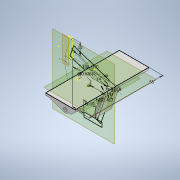
# Autodesk Inventor part: Capping_RotationAnchor
Saved by Autodesk Inventor 2022 (Build 260153000, 153)
## iProperties
Created: 2024-05-05
Part Number: Capping_RotationAnchor
Material: Generic
Document SubType Name: Modeling
Designer: raphael.hauk
Density: 1 g/cm^3
Appearance: Default
Author: raphael.hauk
Autodesk Inventor part; units mm, degrees
ref_plane "YZ Plane" through (0, 0, 0) normal (1, 0, 0) x (0, 1, 0)
ref_plane "XZ Plane" through (0, 0, 0) normal (0, 1, 0) x (-1, 0, 0)
ref_plane "XY Plane" through (0, 0, 0) normal (0, 0, 1) x (1, 0, 0)
ref_plane "Work Plane6" through (7.98, 0, 4.3086) normal (0, 0, 1) x (1, 0, 0)
sketch "Sketch1" plane through (0, 0, 0) normal (0, 0, 1) x (1, 0, 0)
  line L0 (7.98, 8) -> (7.98, -8) projected
  line L1 (7.98, 8) -> (3.98, 8) projected
  line L2 (3.98, -8) -> (3.98, 8) projected
  line L3 (7.98, -8) -> (3.98, -8) projected
  point P0 (0, 0)
  point P1 (21.25, -8.826)
  constraints: 2 other
sketch "Sketch2" plane through (0, 0, 0) normal (0, 0, 1) x (1, 0, 0)
  line L0 (17.98, -43.252) -> (33.98, -43.252)
  line L1 (33.98, -43.252) -> (33.98, -47.252)
  line L2 (33.98, -47.252) -> (17.98, -47.252)
  line L3 (17.98, -47.252) -> (17.98, -43.252)
  line L4 (3.98, -8) -> (3.98, 8) construction
  line L5 (7.98, 8) -> (3.98, 8) construction
  line L6 (7.98, 8) -> (7.98, -8) construction
  line L7 (7.98, -8) -> (3.98, -8) construction
  line L8 (38.606, -12.626) -> (7.98, -2) construction
  line L9 (27.98, -43.252) -> (38.606, -12.626) construction
  arc A0 (7.98, 8) -> (17.98, -43.252) centre (38.606, -12.626) ccw construction
  line L10 (21.25, -8.826) -> (0, -8.826) construction
  line L11 (8.9996, 2.9386) -> (40.245, -7.9022)
  line L12 (40.245, -7.9022) -> (36.967, -17.3498)
  line L13 (36.967, -17.3498) -> (5.7217, -6.5089)
  line L14 (5.7217, -6.5089) -> (8.9996, 2.9386)
  line L15 (8.9996, 2.9386) -> (36.967, -17.3498) construction
  line L16 (40.245, -7.9022) -> (5.7217, -6.5089) construction
  line L17 (38.606, -12.626) -> (27.98, -43.252)
  line L18 (27.98, -43.252) -> (32.7038, -44.891)
  line L19 (32.7038, -44.891) -> (43.3298, -14.265)
  line L20 (43.3298, -14.265) -> (38.606, -12.626)
  point P0 (34.0169, -25.8525)
  point P1 (25.3795, -8.0369)
  point P2 (22.9833, -7.2056)
  point P3 (7.98, 0)
  dimension "d0" = 10
  dimension "d3" = 10
  dimension "d5" = 10
  dimension "d6" = 32.417
  dimension "d7" = 32.417
  dimension "d8" = 3.8
  dimension "d9" = 30.626
  dimension "d26" = 14
  dimension "d27" = 14
  dimension "d44" = 10
  dimension "d47" = 5
  constraints: 34 end point, 7 parallel, 6 point on line, 5 perpendicular, 4 midpoint, 2 horizontal, 2 point on circle, 1 centre point, 1 coincident, 1 collinear
  measures "d0" distance between parallel lines of L3 L6
  measures "d3" distance of L5.start L8.end
  measures "d5" distance of L0.start L9.start
  measures "d6" distance of L8.start L8.end
  measures "d7" distance of L9.start L8.start
  measures "d8" distance from line of L17.start L10
  measures "d9" distance from line of L6 L17.start
  measures "d26" distance of point (25.379, -8.037) L17.start
  measures "d27" distance of point (34.017, -25.853) L17.start
  measures "d44" distance of L11.end L12.end
  measures "d47" distance of L19.end L17.start
ref_plane "Work Plane1" through (18.228, -8.826, 23.9001) normal (0, -1, 0) x (0, 0, -1)
sketch "Sketch3" plane through (18.228, -8.826, 23.9001) normal (0, -1, 0) x (0, 0, -1)
  circle A0 centre (11.5, 16.822) radius 1.45 construction
  circle A1 centre (26.5, 16.822) radius 1.45 construction
  circle A2 centre (11.5, 6.822) radius 1.45 construction
  circle A3 centre (26.5, 6.822) radius 1.45 construction
  line L0 (-12.9085, 2.822) -> (52.0915, 2.822)
  line L1 (52.0915, 2.822) -> (52.0915, 28.822)
  line L2 (52.0915, 28.822) -> (-12.9085, 28.822)
  line L3 (-12.9085, 28.822) -> (-12.9085, 2.822)
  line L4 (19.5915, -18.302) -> (19.5915, 38.076) construction
  point P0 (23.9001, -18.228)
  dimension "d10" = 12
  dimension "d11" = 4
  dimension "d55" = 65
  constraints: 10 end point, 2 parallel, 1 horizontal, 1 perpendicular, 1 vertical, 3 other
  measures "d10" distance from line of L2 A0.centre
  measures "d11" distance from line of L0 A2.centre
  measures "d55" distance of L1.end L2.end
extrude "Extrusion1" add sketch "Sketch3" along normal blind 2
ref_plane "Work Plane3" through (18.228, -12.826, 23.9001) normal (0, -1, 0) x (1, 0, 0)
sketch "Sketch4" plane through (18.228, -12.826, 23.9001) normal (0, -1, 0) x (1, 0, 0)
  point P0 (-18.228, -23.9001)
  point P1 (6.822, -11.5)
  point P2 (6.822, -26.5)
  point P3 (16.822, -11.5)
  point P4 (16.822, -26.5)
sketch "Sketch5" plane through (29.03, -8.826, 4.3086) normal (0, 0, 1) x (1, 0, 0)
  circle A0 centre (9.576, -3.8) radius 1.5
  line L0 (-7.98, -2) -> (18.02, -2) projected
  arc A1 (8.5926, -6.6343) -> (12.4266, -4.7349) centre (9.576, -3.8) ccw
  line L1 (7.937, -8.5238) -> (-23.3083, 2.3171) construction
  line L2 (7.937, -8.5238) -> (-8.6356, -2.7737) construction
  line L3 (-8.6356, -2.7737) -> (-7.98, -0.8842) construction
  line L4 (-7.98, -0.8842) -> (8.5926, -6.6343) construction
  line L5 (8.5926, -6.6343) -> (7.937, -8.5238) construction
  line L6 (-7.98, -2) -> (-7.98, -0.8842)
  line L7 (-7.98, -0.8842) -> (8.5926, -6.6343)
  line L8 (3.6738, -36.065) -> (14.2998, -5.439) construction
  line L9 (14.2998, -5.439) -> (8.5497, -22.0116) construction
  line L10 (8.5497, -22.0116) -> (6.6602, -21.356) construction
  line L11 (6.6602, -21.356) -> (12.4103, -4.7834) construction
  line L12 (12.4103, -4.7834) -> (14.2998, -5.439)
  arc A2 (8.5926, -6.6343) -> (12.4103, -4.7834) centre (9.576, -3.8) ccw construction
  line L13 (14.2998, -5.439) -> (18.02, -2)
  point P0 (-29.03, 8.826)
  point P1 (12.4103, -4.7834)
  point P2 (-4.7641, -2)
  dimension "d21" = 3
  dimension "d46" = 2
  constraints: 22 end point, 5 equal length, 4 perpendicular, 4 point on circle, 4 point on line, 3 centre point, 3 coincident, 1 tangent, 1 vertical
  measures "d21" diameter of A0
  measures "d46" distance between parallel lines of L1 L4
extrude "Extrusion2" add sketch "Sketch5" along normal mid plane 65 contours L0 L13 L12 A1 L7
ref_plane "Work Plane5" through (47.05, -8.826, 4.3086) normal (0, 0, -1) x (-1, 0, 0)
sketch "Sketch7" plane through (47.05, -8.826, 4.3086) normal (0, 0, -1) x (-1, 0, 0)
  line L0 (0, -2) -> (7.4703, -22.7055)
  line L1 (7.4703, -22.7055) -> (9.4703, -22.0116)
  line L2 (3.7202, -5.439) -> (9.4703, -22.0116) construction
  line L3 (0, 0) -> (0, -2) construction
  line L4 (0, -2) -> (3.7202, -5.439)
  line L5 (9.4703, -22.0116) -> (3.7202, -5.439)
  line L6 (0, -2) -> (3.7202, -5.439) projected
  line L7 (0, -2) -> (0, -7.9648)
  line L8 (0, -7.9648) -> (7.4703, -22.7055)
  point P0 (47.05, 8.826)
  point P1 (0, -2)
  dimension "d51" = 2
  constraints: 12 end point, 1 coincident, 1 collinear, 1 perpendicular, 1 vertical
  measures "d51" horizontal distance of L0.end L1.end
extrude "Extrusion3" add sketch "Sketch7" along normal mid plane 14 contours L4 L5 L1 L0
hole "Hole1" at (35.05, -12.826, 12.4001) at (35.05, -12.826, -2.5999) direction (0, 1, 0) diameter 2.6 end through all start extended yes counterbore diameter 5.5 counterbore depth 2 clearance for "Socket Head Cap Screw ISO 4762" size "M2.5" standard "ISO"
fillet "Fillet1" radius 1 2 edges at (45.1899, -12.5455, 11.3086) (45.1899, -12.5455, -2.6914)
sketch "Sketch8" plane through (37.6226, -15.4603, -28.1914) normal (-0.3277907, -0.9447504, 0) x (0.9447504, -0.3277907, 0)
  circle A0 centre (-8, 32.5) radius 5
  line L0 (32.3377, 32.5) -> (-58.7333, 32.5) projected
  line L1 (0, 26.5631) -> (0, 39.6199) projected
  point P0 (-40.6117, 28.1914)
  dimension "d56" = 10
  dimension "d57" = 8
  constraints: 1 centre point, 1 point on line
  measures "d56" diameter of A0
  measures "d57" distance from line of A0.centre L1
extrude "Extrusion4" cut sketch "Sketch8" against normal blind 1
sketch "Sketch9" plane through (37.5797, -30.8376, -2.6914) normal (-0.9447504, 0.3277907, 0) x (0, 0, 1)
  circle A0 centre (7, 9.5418) radius 5
  line L0 (7, -42.3865) -> (7, 53.4932) projected
  line L1 (15, 17.5418) -> (-1, 17.5418) projected
  point P0 (2.6914, 16.8155)
  dimension "d60" = 10
  dimension "d61" = 8
  constraints: 1 centre point, 1 point on line
  measures "d60" diameter of A0
  measures "d61" distance from line of A0.centre L1
extrude "Extrusion5" cut sketch "Sketch9" against normal blind 1
equation "\"d5\" = d3"
equation "\"d7\" = d6"
equation "\"d27\" = d26"
equation "\"d47\" = 0.5 * d44"
body "Solid1"
